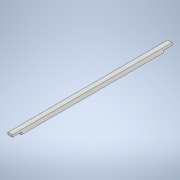
# Autodesk Inventor part: door top
Saved by Autodesk Inventor 2020 (Build 240168000, 168)
## iProperties
Created: 2020-05-09
Part Number: door top
Material: Generic
Document SubType Name: Modeling
Designer: kolbe
Density: 1 g/cm^3
Appearance: Default
Author: kolbe
Autodesk Inventor part; units mm, degrees
ref_plane "YZ Plane" through (0, 0, 0) normal (1, 0, 0) x (0, 1, 0)
ref_plane "XZ Plane" through (0, 0, 0) normal (0, 1, 0) x (-1, 0, 0)
ref_plane "XY Plane" through (0, 0, 0) normal (0, 0, 1) x (1, 0, 0)
sketch "Sketch1" plane through (0, 0, 0) normal (1, 0, 0) x (0, 1, 0)
  line L0 (0, 0) -> (12.7, 0)
  line L1 (12.7, 0) -> (12.7, -901.7)
  line L2 (12.7, -901.7) -> (0, -901.7)
  line L3 (0, -901.7) -> (0, -850.9)
  line L4 (0, -850.9) -> (-12.7, -850.9)
  line L5 (-12.7, -850.9) -> (-12.7, -50.8)
  line L6 (-12.7, -50.8) -> (0, -50.8)
  line L7 (0, -50.8) -> (0, 0)
  dimension "d3" = 12.7
  dimension "d4" = 901.7
  dimension "d5" = 12.7
  dimension "d6" = 50.8
  dimension "d7" = 12.7
  dimension "d8" = 800.1
  constraints: 16 end point, 5 perpendicular, 1 horizontal, 1 parallel, 1 point on line
  measures "d3" distance of L0.start L0.end
  measures "d4" distance of L0.end L1.end
  measures "d5" distance of L1.end L2.end
  measures "d6" distance of L2.end L3.end
  measures "d7" distance of L3.end L4.end
  measures "d8" distance of L4.end L5.end
extrude "Extrusion1" add sketch "Sketch1" along normal mid plane 25.4
body "Solid1"
